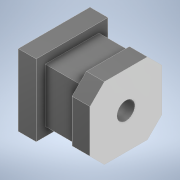
# Autodesk Inventor part: Servo Motor
Saved by Autodesk Inventor 2021 (Build 250183000, 183)
## iProperties
Created: 2021-03-24
Part Number: Servo Motor
Material: Generic
Document SubType Name: Modeling
Designer: calst
Density: 1 g/cm^3
Appearance: Smooth - Black
Author: calst
Autodesk Inventor part; units mm, degrees
ref_plane "YZ Plane" through (0, 0, 0) normal (1, 0, 0) x (0, 1, 0)
ref_plane "XZ Plane" through (0, 0, 0) normal (0, 1, 0) x (-1, 0, 0)
sketch "Sketch1" plane through (0, 0, 0) normal (1, 0, 0) x (0, 1, 0)
  circle A0 centre (0, 0) radius 2.5
  line L0 (-10, 10) -> (10, 10)
  line L1 (10, 10) -> (10, -10)
  line L2 (10, -10) -> (-10, -10)
  line L3 (-10, -10) -> (-10, 10)
  line L4 (-10, 10) -> (10, -10) construction
  line L5 (10, 10) -> (-10, -10) construction
  dimension "d0" = 5
  dimension "d1" = 20
  dimension "d2" = 20
  constraints: 12 end point, 2 midpoint, 2 parallel, 1 centre point, 1 coincident, 1 horizontal, 1 perpendicular
  measures "d0" diameter of A0
  measures "d1" distance of L0.start L0.end
  measures "d2" distance of L0.end L1.end
extrude "Extrusion1" add sketch "Sketch1" along normal blind 20
ref_plane "Work Plane1" through (15, 0, 0) normal (1, 0, 0) x (0, 0, -1)
sketch "Sketch2" plane through (15, 0, 0) normal (1, 0, 0) x (0, 0, -1)
  line L0 (10, -10) -> (10, 10) projected
  line L1 (-10, -10) -> (10, -10)
  line L2 (10, -10) -> (10, 10)
  line L3 (10, 10) -> (-10, 10)
  line L4 (-10, 10) -> (-10, -10)
  line L5 (-10, -10) -> (10, 10) construction
  line L6 (10, -10) -> (-10, 10) construction
  line L7 (-7.5, -7.5) -> (7.5, -7.5)
  line L8 (7.5, -7.5) -> (7.5, 7.5)
  line L9 (7.5, 7.5) -> (-7.5, 7.5)
  line L10 (-7.5, 7.5) -> (-7.5, -7.5)
  line L11 (-7.5, -7.5) -> (7.5, 7.5) construction
  line L12 (7.5, -7.5) -> (-7.5, 7.5) construction
  point P0 (0, 0)
  dimension "d6" = 15
  dimension "d7" = 15
  constraints: 24 end point, 4 midpoint, 4 parallel, 2 horizontal, 2 perpendicular
  measures "d6" distance of L9.end L8.end
  measures "d7" distance of L9.end L7.start
extrude "Extrusion2" cut sketch "Sketch2" against normal blind 10
chamfer "Chamfer1" distance 4 angle 45 4 edges at (17.5, 10, 10) (17.5, 10, -10) (17.5, -10, -10) (17.5, -10, 10)
body "Solid1"
